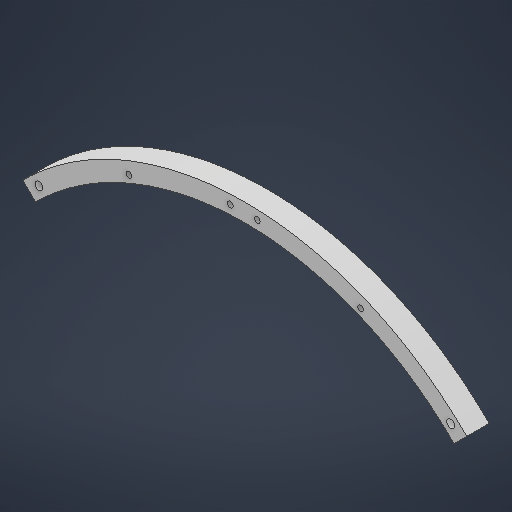
# Autodesk Inventor part: 组合
Saved by Autodesk Inventor 2025 (Build 290162000, 162)
## iProperties
Created: 2025-02-22
Part Number: 组合
Material: 常规
Document SubType Name: Modeling
Designer: XH
Density: 1 g/cm^3
Appearance: 默认
Author: XH
Autodesk Inventor part; units mm, degrees
ref_plane "YZ Plane" through (0, 0, 0) normal (1, 0, 0) x (0, 1, 0)
ref_plane "XZ Plane" through (0, 0, 0) normal (0, 1, 0) x (-1, 0, 0)
ref_plane "XY Plane" through (0, 0, 0) normal (0, 0, 1) x (1, 0, 0)
sketch "草图1" plane through (0, 0, 0) normal (0, 0, 1) x (1, 0, 0)
  circle A0 centre (0, 0) radius 140
  circle A1 centre (0, 0) radius 132
  line L0 (0, 140) -> (0, -140)
  line L1 (140, 0) -> (-140, 0)
  line L2 (-98.9949, 98.9949) -> (98.9949, -98.9949)
  line L3 (98.9949, 98.9949) -> (-98.9949, -98.9949)
  point P0 (-93.3381, 93.3381)
  point P1 (93.3381, 93.3381)
  dimension "d0" = 280
  dimension "d1" = 8
  dimension "d2" = 90
  dimension "d5" = 45
  constraints: 8 end point, 4 coincident, 4 point on circle, 3 midpoint, 2 centre point, 9 other
  measures "d0" diameter of A0
  measures "d1" radial gap between concentric circles of A1 A0
  measures "d2" angle of L0 L1
extrude "拉伸1" add sketch "草图1" along normal blind 10 contours L3 A1 L0 A0 | L0 A1 L2 A0 picked at (81.3579, 110.3999) picked at (-77.3338, 113.2551)
sketch "草图2" plane through (0, 0, 0) normal (0, 0, -1) x (-1, 0, 0)
  circle A0 centre (0, 0) radius 136
  arc A1 (93.3381, 93.3381) -> (-93.3381, 93.3381) centre (0, 0) ccw projected
  arc A2 (98.9949, 98.9949) -> (-98.9949, 98.9949) centre (0, 0) ccw projected
  circle A3 centre (91.8302, 100.3155) radius 1.75
  line L0 (98.9949, 98.9949) -> (93.3381, 93.3381) projected
  line L1 (0, 140) -> (0, 106.7843)
  circle A4 centre (-91.8302, 100.3155) radius 1.75
  dimension "d9" = 4
  dimension "d11" = 3.5
  dimension "d12" = 6
  constraints: 2 centre point, 2 end point, 1 coincident, 1 point on circle, 1 symmetric about line, 1 vertical, 4 other
  measures "d11" diameter of A3
  measures "d12" distance from line of A3.centre L0
extrude "拉伸2" cut sketch "草图2" against normal blind 29.25 contours A4 A0 | A0 A4 | A3 A0 | A0 A3
sketch "草图3" plane through (0, 0, 0) normal (0, 0, -1) x (-1, 0, 0)
  circle A0 centre (6.4504, 135.8469) radius 1.5
  circle A1 centre (-100.3405, 91.803) radius 1.5 projected
  circle A2 centre (-100.3405, 91.803) radius 1.5 projected
  circle A3 centre (-5.5864, 135.8852) radius 1.5 projected
  circle A4 centre (6.4504, 135.8469) radius 1.25
  circle A5 centre (-5.5864, 135.8852) radius 1.25
  point P0 (0, 0)
  dimension "d27" = 2.5
  dimension "d28" = 2.5
  constraints: 3 centre point, 2 coincident, 2 other
  measures "d27" diameter of A4
  measures "d28" diameter of A5
extrude "拉伸3" cut sketch "草图3" against normal blind 29.25 contours A4 | A5
sketch "草图4" plane through (0, 0, 10) normal (0, 0, 1) x (1, 0, 0)
  line L0 (0, 0) -> (-63.3975, 153.0551)
  line L1 (0, 0) -> (0, 175.6772)
  line L2 (0, 0) -> (-105.4105, 105.4105)
  line L3 (-98.9949, 98.9949) -> (-93.3381, 93.3381) projected
  circle A0 centre (0, 0) radius 135.032
  circle A1 centre (-51.6745, 124.7533) radius 1.5
  circle A2 centre (51.6745, 124.7533) radius 1.5
  circle A3 centre (-51.6745, 124.7533) radius 1.25
  circle A4 centre (51.6745, 124.7533) radius 1.25
  dimension "d23" = 270.064
  dimension "d21" = 22.5
  dimension "d22" = 22.5
  dimension "d24" = 3
  dimension "d33" = 2.5
  dimension "d34" = 2.5
  constraints: 6 end point, 4 centre point, 3 coincident, 1 collinear, 1 point on line, 1 symmetric about line, 1 vertical, 4 other
  measures "d21" angle of L0 L1
  measures "d22" angle of L0 L2
  measures "d24" diameter of A1
  measures "d33" diameter of A3
  measures "d34" diameter of A4
extrude "拉伸4" cut sketch "草图4" against normal blind 10 contours A3 A0 L0 | L0 A0 A3 | A0 A3 L0 | L0 A3 A0 | A4 A0 | A0 A4
thread "螺纹1" size "M3x0.5" class "6H" standard "ANSI Metric M Profile" full length
thread "螺纹2" size "M3x0.5" class "6H" standard "ANSI Metric M Profile" full length
thread "螺纹3" size "M3x0.5" class "6H" standard "ANSI Metric M Profile" full length
thread "螺纹4" size "M3x0.5" class "6H" standard "ANSI Metric M Profile" full length
sketch "草图7" plane through (0, 0, 0) normal (0, 0, -1) x (-1, 0, 0)
  circle A0 centre (-91.8302, 100.3155) radius 1.75 projected
  circle A1 centre (-91.8302, 100.3155) radius 2.75
  point P0 (0, 0)
  dimension "d39" = 5.5
  constraints: 1 centre point, 1 coincident
  measures "d39" diameter of A1
extrude "拉伸5" cut sketch "草图7" against normal blind 6 contours A0 | A1
mirror "镜像1" about plane through (0, 0, 0) normal (1, 0, 0) of "拉伸5"
